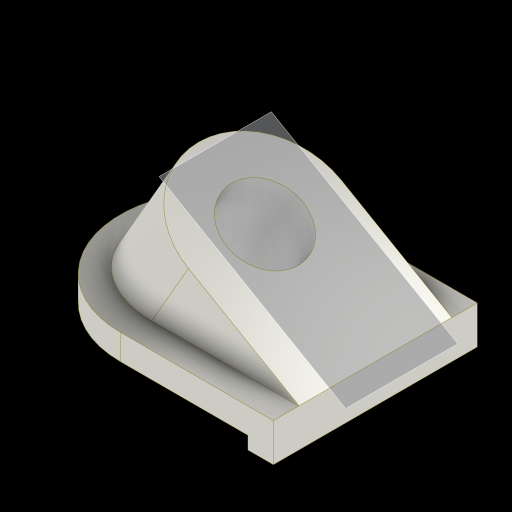
# Autodesk Inventor part: ANS9-3-BK
Saved by Autodesk Inventor 2024 (Build 280153000, 153)
## iProperties
Created: 2023-10-29
Part Number: ANS9-3-BK
Material: Silver
Document SubType Name: Modeling
Designer: bennk
Density: 10.49 g/cm^3
Appearance: Silver
Mass: 3074.21 g
Surface Area: 412.735 cm^2
Volume: 293.061 cm^3
Author: bennk
Autodesk Inventor part; units mm, degrees
ref_plane "YZ Plane" through (0, 0, 0) normal (1, 0, 0) x (0, 1, 0)
ref_plane "XZ Plane" through (0, 0, 0) normal (0, 1, 0) x (-1, 0, 0)
ref_plane "XY Plane" through (0, 0, 0) normal (0, 0, 1) x (1, 0, 0)
sketch "Sketch1" plane through (0, 0, 0) normal (0, 1, 0) x (-1, 0, 0)
  circle A0 centre (0, 0) radius 50.8
  line L0 (0, 50.8) -> (-76.2, 50.8)
  line L1 (-76.2, 50.8) -> (-76.2, -50.8)
  line L2 (-76.2, -50.8) -> (0, -50.8)
  line L3 (0, -50.8) -> (0, 50.8)
  dimension "d0" = 101.6
  dimension "d1" = 76.2
  constraints: 8 end point, 2 parallel, 2 point on circle, 1 centre point, 1 coincident, 1 horizontal, 1 midpoint, 1 perpendicular
  measures "d0" diameter of A0
  measures "d1" distance of L2.end L1.end
extrude "BASE" add sketch "Sketch1" against normal blind 12.7
sketch "Sketch2" plane through (76.2, 0, 50.8) normal (1, 0, 0) x (0, 0, -1)
  line L0 (101.6, -12.7) -> (0, -12.7) projected
  line L1 (0, -12.7) -> (101.6, -12.7)
  line L2 (101.6, -12.7) -> (101.6, -19.05)
  line L3 (101.6, -19.05) -> (0, -19.05)
  line L4 (0, -19.05) -> (0, -12.7)
  point P0 (50.8, 0)
  dimension "d4" = 6.35
  constraints: 8 end point, 2 parallel, 1 horizontal, 1 perpendicular, 1 point on line
  measures "d4" distance of L3.end L0.end
extrude "LIP" add sketch "Sketch2" against normal blind 12.7
ref_plane "ANGLE PLANE" through (76.2, 0, 50.8) normal (0.5, 0.8660254, 0) x (0, 0, -1)
sketch "Sketch3" plane through (76.2, 0, 50.8) normal (0.5, 0.8660254, 0) x (0, 0, -1)
  line L0 (0, 0) -> (101.6, 0) projected
  line L1 (12.7, 0) -> (88.9, 0)
  line L2 (88.9, 0) -> (88.9, 63.5)
  line L3 (88.9, 63.5) -> (12.7, 63.5)
  line L4 (12.7, 63.5) -> (12.7, 0)
  circle A0 centre (50.8, 63.5) radius 38.1
  circle A1 centre (50.8, 63.5) radius 19.05
  point P0 (50.8, 65.9911)
  point P1 (12.7, 63.5)
  point P2 (88.9, 0)
  dimension "d8" = 76.2
  dimension "d10" = 38.1
  dimension "d11" = 63.5
  dimension "d12" = 12.7
  constraints: 8 end point, 2 centre point, 2 parallel, 1 coincident, 1 horizontal, 1 midpoint, 1 perpendicular, 1 point on line, 1 tangent
  measures "d8" distance between parallel lines of L2 L4
  measures "d10" diameter of A1
  measures "d11" distance of L3.end L1.start
  measures "d12" distance from line of L0.end L2
extrude "AGNLED FACE" add sketch "Sketch3" against normal through all
extrude "HOLE" cut sketch "Sketch3" against normal through all contours A1 L3 | L3 A1
body "Solid1"
